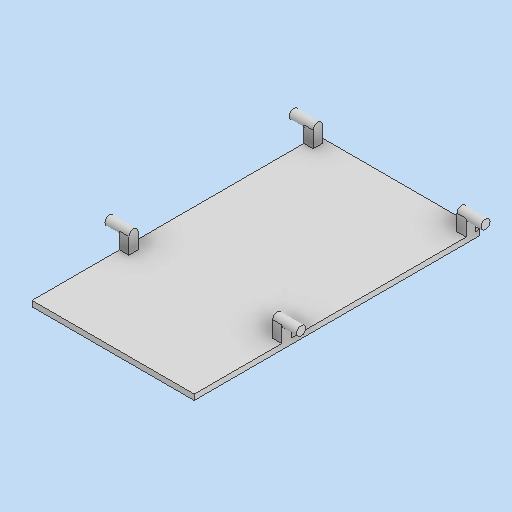
# Autodesk Inventor part: lift plate
Saved by Autodesk Inventor 2026 (Build 300175000, 175)
## iProperties
Created: 2026-02-03
Part Number: lift plate
Material: Generic
Document SubType Name: Modeling
Designer: mones
Density: 1 g/cm^3
Appearance: Default
Author: mones
Autodesk Inventor part; units mm, degrees
ref_plane "YZ Plane" through (0, 0, 0) normal (1, 0, 0) x (0, 1, 0)
ref_plane "XZ Plane" through (0, 0, 0) normal (0, 1, 0) x (-1, 0, 0)
ref_plane "XY Plane" through (0, 0, 0) normal (0, 0, 1) x (1, 0, 0)
sketch "Sketch1" plane through (0, 0, 0) normal (0, 1, 0) x (-1, 0, 0)
  line L0 (44, 50) -> (44, -50)
  line L1 (44, -50) -> (-44, -50)
  line L2 (-44, -50) -> (-44, 50)
  line L3 (-44, 50) -> (44, 50)
  line L4 (44, 50) -> (-44, -50) construction
  line L5 (44, -50) -> (-44, 50) construction
  line L6 (44, -50) -> (44, -55)
  line L7 (-44, -50) -> (-44, -55)
  line L8 (-44, -55) -> (44, -55)
  line L9 (44, 50) -> (44, 100)
  line L10 (-44, 50) -> (-44, 100)
  line L11 (-44, 100) -> (44, 100)
  point P0 (0, 0)
  dimension "d0" = 100
  dimension "d1" = 88
  dimension "d2" = 5
  dimension "d3" = 5
  dimension "d4" = 50
  dimension "d5" = 50
  constraints: 24 end point, 3 vertical, 2 midpoint, 2 parallel, 2 perpendicular, 1 point on line
  measures "d0" distance of L0.start L0.end
  measures "d1" distance of L0.end L1.end
  measures "d2" distance of L0.end L6.end
  measures "d3" distance of L1.end L7.end
  measures "d4" distance of L0.start L9.end
  measures "d5" distance of L2.end L10.end
extrude "Extrusion1" add sketch "Sketch1" along normal blind 3
sketch "Sketch2" plane through (0, 3, 0) normal (0, 1, 0) x (1, 0, 0)
  line L0 (-44, 55) -> (-44, -100) projected
  line L1 (-44, -100) -> (44, -100) projected
  line L2 (44, -100) -> (44, 55) projected
  line L3 (44, 55) -> (-44, 55) projected
  line L4 (-44, -100) -> (-44, -50)
  line L5 (-44, -50) -> (-44, 50)
  line L6 (-44, 50) -> (44, 50)
  line L7 (44, 50) -> (44, -50)
  line L8 (44, -50) -> (44, -100)
  line L9 (44, -50) -> (-44, -50)
  line L10 (-44, -50) -> (-39, -50)
  line L11 (-39, -50) -> (-39, -47.5)
  line L12 (-44, -52.5) -> (-39, -52.5)
  line L13 (-39, -52.5) -> (-39, -47.5)
  line L14 (-39, -47.5) -> (-44, -47.5)
  line L15 (-44, -47.5) -> (-44, -52.5)
  line L16 (-44, -52.5) -> (-39, -47.5) construction
  line L17 (-39, -52.5) -> (-44, -47.5) construction
  line L18 (44, -50) -> (41.5, -50)
  line L19 (41.5, -50) -> (41.5, -47.5)
  line L20 (44, 50) -> (41.5, 50)
  line L21 (41.5, 50) -> (41.5, 52.5)
  line L22 (-44, 50) -> (-41.5, 50)
  line L23 (-41.5, 50) -> (-41.5, 52.5)
  line L24 (39, -52.5) -> (39, -47.5)
  line L25 (39, -47.5) -> (44, -47.5)
  line L26 (44, -47.5) -> (44, -52.5)
  line L27 (44, -52.5) -> (39, -52.5)
  line L28 (39, -52.5) -> (44, -47.5) construction
  line L29 (39, -47.5) -> (44, -52.5) construction
  line L30 (39, 47.5) -> (39, 52.5)
  line L31 (39, 52.5) -> (44, 52.5)
  line L32 (44, 52.5) -> (44, 47.5)
  line L33 (44, 47.5) -> (39, 47.5)
  line L34 (39, 47.5) -> (44, 52.5) construction
  line L35 (39, 52.5) -> (44, 47.5) construction
  line L36 (-39, 47.5) -> (-44, 47.5)
  line L37 (-44, 47.5) -> (-44, 52.5)
  line L38 (-44, 52.5) -> (-39, 52.5)
  line L39 (-39, 52.5) -> (-39, 47.5)
  line L40 (-39, 47.5) -> (-44, 52.5) construction
  line L41 (-44, 47.5) -> (-39, 52.5) construction
  point P0 (-41.5, -50)
  dimension "d8" = 50
  dimension "d9" = 100
  dimension "d10" = 5
  dimension "d11" = 2.5
  dimension "d12" = 2.5
  dimension "d13" = 2.5
  dimension "d14" = 2.5
  dimension "d15" = 2.5
  dimension "d16" = 2.5
  constraints: 76 end point, 11 parallel, 10 perpendicular, 9 midpoint, 8 point on line, 1 collinear, 1 horizontal
  measures "d8" distance of L0.end L4.end
  measures "d9" distance of L4.end L5.end
  measures "d10" distance of L4.end L10.end
  measures "d11" distance of L10.end L11.end
  measures "d12" distance of L7.end L18.end
  measures "d13" distance of L18.end L19.end
  measures "d14" distance of L6.end L20.end
  measures "d15" distance of L20.end L21.end
  measures "d16" distance of L5.end L22.end
extrude "Extrusion2" add sketch "Sketch2" along normal blind 8.73 contours L38 L23 L6 L0 | L6 L39 L36 L0 | L38 L39 L6 L23 | L2 L6 L21 L31 | L2 L33 L30 L6 | L21 L6 L30 L31 | L14 L11 L9 L0 | L9 L13 L12 L0 | L2 L9 L19 L25 | L2 L27 L24 L9 | L19 L9 L24 L25
sketch "Sketch3" plane through (44, 0, 100) normal (1, 0, 0) x (0, 0, -1)
  line L0 (147.5, 11.73) -> (152.5, 11.73) projected
  circle A0 centre (150, 11.73) radius 2.5
  constraints: 1 horizontal alignment, 1 midpoint, 2 other
sketch "Sketch4" plane through (44, 0, 100) normal (1, 0, 0) x (0, 0, -1)
  line L0 (47.5, 11.73) -> (52.5, 11.73) projected
  circle A0 centre (50, 11.73) radius 2.5
  constraints: 1 horizontal alignment, 1 midpoint, 2 other
extrude "Extrusion3" add sketch "Sketch4" against normal blind 5
extrude "Extrusion4" add sketch "Sketch3" against normal blind 5
sketch "Sketch5" plane through (-44, 0, -55) normal (-1, 0, 0) x (0, 0, 1)
  line L0 (2.5, 11.73) -> (7.5, 11.73) projected
  circle A0 centre (5, 11.73) radius 2.5
  constraints: 1 midpoint, 3 other
sketch "Sketch6" plane through (-44, 0, -55) normal (-1, 0, 0) x (0, 0, 1)
  line L0 (102.5, 11.73) -> (107.5, 11.73) projected
  circle A0 centre (105, 11.73) radius 2.5
  constraints: 1 midpoint, 3 other
extrude "Extrusion5" add sketch "Sketch5" against normal blind 5 contours A0 L0 picked at (5.695, 12.8693)
extrude "Extrusion6" add sketch "Sketch6" against normal blind 5 contours A0 L0 picked at (105.7192, 12.6699)
sketch "Sketch7" plane through (-44, 0, -55) normal (-1, 0, 0) x (0, 0, 1)
  arc A0 (7.5, 11.73) -> (2.5, 11.73) centre (5, 11.73) ccw projected
  arc A1 (107.5, 11.73) -> (102.5, 11.73) centre (105, 11.73) ccw projected
  circle A2 centre (5, 11.73) radius 2.5
  circle A3 centre (105, 11.73) radius 2.5
  constraints: 2 coincident, 6 other
extrude "Extrusion7" add sketch "Sketch7" along normal blind 8
sketch "Sketch8" plane through (44, 0, 100) normal (1, 0, 0) x (0, 0, -1)
  arc A0 (52.5, 11.73) -> (47.5, 11.73) centre (50, 11.73) ccw projected
  arc A1 (152.5, 11.73) -> (147.5, 11.73) centre (150, 11.73) ccw projected
  circle A2 centre (50, 11.73) radius 2.5
  circle A3 centre (150, 11.73) radius 2.5
  constraints: 2 coincident, 6 other
extrude "Extrusion8" add sketch "Sketch8" along normal blind 8
body "Solid1"
